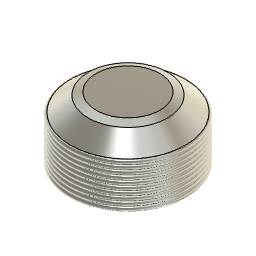
PUMP THING (Autodesk Fusion 360 design; units mm, degrees)
Autodesk Fusion 360 part; units mm, degrees
note: some values were not read from the file. Set by a fixed rule: which sketch regions a step uses.
sketch "Sketch1" plane through (0, 0, 0) normal (0, 1, 0) x (1, 0, 0)
  line L0 (0, 0) -> (82.55, 0)
  line L1 (82.55, 0) -> (82.55, -6.35)
  line L2 (82.55, -6.35) -> (0, -6.35)
  line L3 (0, -6.35) -> (0, 0)
  circle A0 centre (82.55, -3.175) radius 3.175
  constraint horizontal L0
  constraint vertical L1
  constraint horizontal L2
  constraint vertical L3
  constraint coincident L0.start L3.end
  constraint midpoint L1 A0.centre
  constraint coincident L0.end A0
revolve "Revolve1" add sketch "Sketch1" angle 360 about axis through (0, 0, 1.75) along (0, 0, 1) makes body 1
extrude "Extrude1" add 1 faces at (-14.0657, -19.729, 6.35) along direction (0, 0, 1) blind 0.0635 on bodies 1 bodies 1
pattern_linear "R-Pattern1" count 10 spacing 6.4911 along (0, 0, 1) of bodies 1 makes body 2 at (21.8202, -3.2889, 6.4911) makes body 3 at (21.8202, -3.2889, 12.9822) makes body 4 at (21.8202, -3.2889, 19.4733) makes body 5 at (21.8202, -3.2889, 25.9644) makes body 6 at (21.8202, -3.2889, 32.4556) makes body 7 at (21.8202, -3.2889, 38.9467) makes body 8 at (21.8202, -3.2889, 45.4378) makes body 9 at (21.8202, -3.2889, 51.9289) makes body 10 at (21.8202, -3.2889, 58.42)
extrude "Extrude2" add 1 faces at (-14.0657, -19.729, 64.8335) along direction (0, 0, 1) blind 25.4 draft -50 on bodies 10 bodies 10
chamfer "Chamfer1" distance 6.35 angle 45 1 faces at (6.9462, -18.7611, 90.2335) on bodies 10
